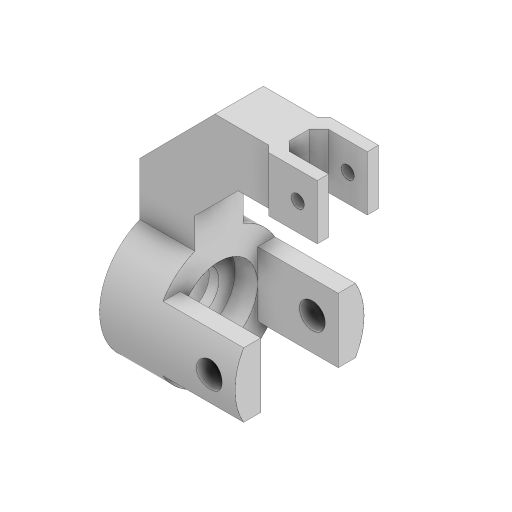
# Autodesk Inventor part: Wheel hub left ver 2
Saved by Autodesk Inventor 2023 (Build 270158000, 158)
## iProperties
Created: 2023-03-21
Part Number: Wheel hub left ver 2
Material: Generic
Document SubType Name: Modeling
Designer: Juyoung Han
Density: 1 g/cm^3
Appearance: Default
Mass: 23.6311 g
Surface Area: 102.719 cm^2
Volume: 23.6311 cm^3
Author: Juyoung Han
Autodesk Inventor part; units mm, degrees
ref_plane "YZ Plane" through (0, 0, 0) normal (1, 0, 0) x (0, 1, 0)
sketch "Sketch1" plane through (0, 0, 0) normal (0, 0, 1) x (1, 0, 0)
  line L0 (0, 7) -> (3, 7)
  line L1 (3, 7) -> (0, 7)
  line L2 (0, 7) -> (0, 12)
  line L3 (0, 12) -> (-7, 12)
  line L4 (-7, 12) -> (-7, 20)
  line L5 (-7, 20) -> (10, 20)
  line L6 (10, 20) -> (10, 12)
  line L7 (10, 12) -> (3, 12)
  line L8 (3, 12) -> (3, 7)
  line L9 (-10.4, 0) -> (13.4, 0) projected
  point P0 (0, 0)
  dimension "d0" = 3
  dimension "d1" = 5
  dimension "d2" = 7
  dimension "d3" = 8
  dimension "d4" = 17
  dimension "d5" = 8
  dimension "d6" = 7
  constraints: 18 end point, 4 perpendicular, 3 horizontal, 1 collinear, 1 point on line
  measures "d0" distance of L0.start L0.end
  measures "d1" distance of L0.start L2.end
  measures "d2" distance of L2.end L3.end
  measures "d3" distance of L3.end L4.end
  measures "d4" distance of L4.end L5.end
  measures "d5" distance of L5.end L6.end
  measures "d6" distance from line of point (0, 0) L0
revolve "Revolution1" add sketch "Sketch1" angle 360 about axis through (-10, 0, 0) along (1, 0, 0)
ref_plane "Work Plane1" through (0, 0, 14) normal (0, 0, 1) x (1, 0, 0)
ref_plane "Work Plane2" through (0, 0, -14) normal (0, 0, 1) x (1, 0, 0)
sketch "Sketch46" plane through (0, 0, 14) normal (0, 0, 1) x (1, 0, 0)
  point P0 (0, 0)
sketch "Sketch47" plane through (0, 0, 0) normal (0, 0, 1) x (1, 0, 0)
  line L0 (0, 0) -> (51.7638, 0) construction
  line L1 (-7, 41.5) -> (-7, 41.6234)
  line L2 (-7, 20) -> (10, 20)
  line L3 (-7, 20) -> (10, 20) projected
  line L4 (0, 0) -> (70.7107, 0) construction
  line L5 (50, 58.5) -> (50, 41.5)
  line L6 (50, 41.5) -> (30, 41.5)
  line L7 (50, 58.5) -> (30, 58.5)
  line L8 (10, -20) -> (10, 20) projected
  line L9 (-7, -20) -> (-7, 20) projected
  line L10 (-7, 20) -> (-7, 35)
  line L11 (-7, 35) -> (16.2804, 58.5)
  line L12 (16.2804, 58.5) -> (30, 58.5)
  line L13 (14.7544, 32.8045) -> (10, 28.0502)
  line L14 (10, 28.0502) -> (10, 20)
  line L15 (-7, 20) -> (10, 20) projected
  line L16 (14.7544, 32.8045) -> (23.4498, 41.5)
  line L17 (23.4498, 41.5) -> (30, 41.5)
  line L18 (0, 0) -> (10, 10)
  constraints: 30 end point, 4 horizontal, 3 perpendicular, 3 point on line, 2 vertical, 1 collinear
extrude "Extrusion42" add sketch "Sketch47" along normal mid plane 15
sketch "Sketch54" plane through (10, 0, 0) normal (1, 0, 0) x (0, 0, -1)
  arc A0 (7.5, 18.5405) -> (-7.5, 18.5405) centre (0, 0) ccw
  line L0 (-7.5, 20) -> (0, 20) projected
  line L1 (7.5, 20) -> (-7.5, 20)
  line L2 (-7.5, 20) -> (-7.5, 18.5405)
  line L3 (7.5, 20) -> (7.5, 18.5405)
  circle A1 centre (0, 0) radius 20 projected
  constraints: 6 end point, 3 point on circle, 1 centre point, 1 coincident, 1 horizontal, 1 parallel, 1 perpendicular
extrude "Extrusion48" add sketch "Sketch54" against normal up to surface (17 mm away) contours A0 L1 L3 | A0 L2 L0
sketch "Sketch55" plane through (10, 18.5405, 7.5) normal (1, 0, 0) x (0, 0, -1)
  line L0 (19.5, -8.5405) -> (19.5, -28.5405)
  line L1 (19.5, -8.5405) -> (24.8205, -8.5405)
  line L2 (19.5, -28.5405) -> (24.8205, -28.5405)
  arc A0 (0, 0) -> (15, 0) centre (7.5, -18.5405) ccw projected
  line L3 (-4.5, -8.5405) -> (-4.5, -28.5405)
  line L4 (-4.5, -8.5405) -> (-9.8205, -8.5405)
  line L5 (-4.5, -28.5405) -> (-9.8205, -28.5405)
  arc A1 (24.8205, -28.5405) -> (24.8205, -8.5405) centre (7.5, -18.5405) ccw
  arc A2 (-9.8205, -8.5405) -> (-9.8205, -28.5405) centre (7.5, -18.5405) ccw
  point P0 (19.5, -18.5405)
  constraints: 12 end point, 5 point on circle, 2 centre point, 1 coincident, 1 horizontal, 1 midpoint, 1 parallel, 1 vertical
extrude "Extrusion49" add sketch "Sketch55" along normal blind 25
sketch "Sketch56" plane through (10, -10, 12) normal (0, 0, -1) x (-1, 0, 0)
  circle A0 centre (-17, 10) radius 4
  line L0 (-25, 0) -> (-25, 20) projected
  point P0 (10, 10)
  point P1 (-25, 10)
  dimension "d298" = 8
  dimension "d299" = 8
  constraints: 1 centre point, 1 midpoint
  measures "d298" diameter of A0
  measures "d299" distance of point (-25, 10) A0.centre
extrude "Extrusion50" cut sketch "Sketch56" along normal through all both and the other way through all
sketch "Sketch57" plane through (23.4498, 41.5, 7.5) normal (0, -1, 0) x (1, 0, 0)
  line L0 (26.5502, -15) -> (26.5502, 0) projected
  line L1 (26.5502, -13.5) -> (11.5502, -13.5)
  line L2 (11.5502, -13.5) -> (11.5502, -1.5)
  line L3 (11.5502, -1.5) -> (26.5502, -1.5)
  line L4 (26.5502, -1.5) -> (26.5502, -13.5)
  point P0 (-23.4498, -7.5)
  point P1 (26.5502, -7.5)
  point P2 (11.5502, -7.5)
  dimension "d302" = 15
  dimension "d303" = 12
  dimension "d304" = 0
  constraints: 8 end point, 2 midpoint, 2 parallel, 1 horizontal, 1 perpendicular, 1 point on line
  measures "d302" distance of L2.end L3.end
  measures "d303" distance of L1.end L2.end
  measures "d304" vertical distance of point (26.55, -7.5) point (11.55, -7.5)
extrude "Extrusion51" cut sketch "Sketch57" against normal through all
sketch "Sketch59" plane through (0, 0, -7.5) normal (0, 0, -1) x (-1, 0, 0)
  point P0 (0, 0)
sketch "Sketch60" plane through (0, 0, -7.5) normal (0, 0, -1) x (-1, 0, 0)
  point P0 (0, 0)
sketch "Sketch62" plane through (16.2804, 58.5, -7.5) normal (0, 1, 0) x (1, 0, 0)
  line L0 (18.7196, -1.5) -> (33.7196, -1.5) projected
  line L1 (0, 0) -> (33.7196, 0) projected
  line L2 (18.7196, 0) -> (33.7196, 0)
  line L3 (33.7196, 0) -> (33.7196, 2)
  line L4 (33.7196, 2) -> (18.7196, 2)
  line L5 (33.7196, -15) -> (0, -15) projected
  line L6 (18.7196, -15) -> (33.7196, -15)
  line L7 (33.7196, -15) -> (33.7196, -17)
  line L8 (33.7196, -17) -> (18.7196, -17)
  line L9 (18.7196, 2) -> (16.7196, 0)
  line L10 (33.7196, 0) -> (7.1694, 0) projected
  line L11 (18.7196, 2) -> (21.548, 2) construction
  line L12 (18.7196, 0) -> (16.7196, 0)
  line L13 (18.7196, -17) -> (16.7196, -15)
  line L14 (18.7196, -15) -> (16.7196, -15)
  point P0 (-16.2804, -7.5)
  point P1 (16.7196, 0)
  dimension "d318" = 2
  dimension "d319" = 2
  dimension "d322" = 135
  constraints: 22 end point, 5 point on line, 3 horizontal, 3 parallel, 2 perpendicular, 1 collinear, 1 equal length
  measures "d318" distance of L3.end L2.end
  measures "d319" distance of L6.end L7.end
  measures "d322" angle of L9 L11
extrude "Extrusion53" add sketch "Sketch62" against normal up to surface (17 mm away)
sketch "Sketch63" plane through (50, 41.5, 6) normal (0, 0, -1) x (-1, 0, 0)
  circle A0 centre (6, 8.5) radius 2
  line L0 (0, 0) -> (0, 17) projected
  point P0 (50, -41.5)
  dimension "d323" = 4
  dimension "d324" = 6
  constraints: 1 centre point
  measures "d323" diameter of A0
  measures "d324" distance from line of L0 A0.centre
extrude "Extrusion54" cut sketch "Sketch63" along normal through all both and the other way through all
sketch "Sketch64" plane through (16.2804, 58.5, 7.5) normal (0, 1, 0) x (1, 0, 0)
  line L0 (18.7196, 1.5) -> (33.7196, 1.5) projected
  line L1 (21.548, 1.5) -> (18.7196, 4.3284)
  line L2 (21.548, 1.5) -> (25.548, 1.5) construction
  line L3 (18.7196, 1.5) -> (18.7196, 13.5) projected
  line L4 (21.548, 1.5) -> (18.7196, 1.5)
  line L5 (18.7196, 13.5) -> (33.7196, 13.5) projected
  line L6 (21.548, 13.5) -> (18.7196, 10.6716)
  line L7 (21.548, 13.5) -> (25.548, 13.5) construction
  line L8 (18.7196, 13.5) -> (18.7196, 1.5) projected
  line L9 (18.7196, 10.6716) -> (18.7196, 13.5)
  line L10 (18.7196, 13.5) -> (21.548, 13.5)
  line L11 (18.7196, 1.5) -> (18.7196, 4.3284)
  point P0 (-16.2804, 7.5)
  point P1 (18.7196, 4.3284)
  dimension "d327" = 4
  dimension "d328" = 135
  dimension "d329" = 0
  dimension "d330" = 135
  dimension "d331" = 4
  dimension "d332" = 0
  constraints: 16 end point, 2 equal length, 2 horizontal, 2 point on line, 1 collinear
  measures "d327" distance of L1.start L1.end
  measures "d328" angle of L2 L1
  measures "d329" distance from line of L1.end L3
  measures "d330" angle of L6 L7
  measures "d331" distance of L6.start L6.end
  measures "d332" distance from line of L3 L6.end
extrude "Extrusion55" add sketch "Sketch64" against normal up to surface (17 mm away)
body "Solid1"
